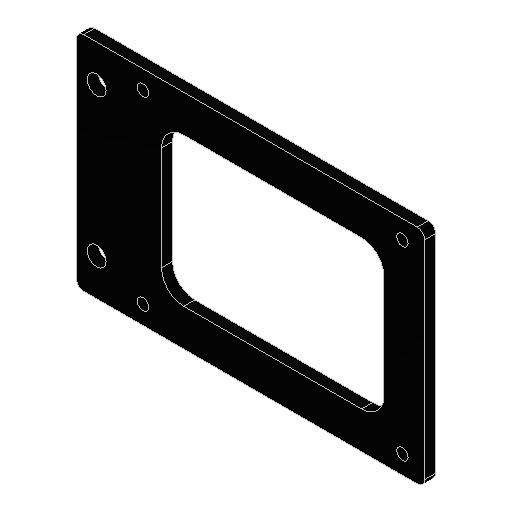
# Autodesk Inventor part: PCB plate
Saved by Autodesk Inventor 2022.4 (Build 264492000, 492)
## iProperties
Category: -
Company: Universiteit van Amsterdam
Created: 2023-09-04
Part Number: PCB plate
Material: ALMg4,5Mn-5083-(D54S)
Document SubType Name: Modeling
Designer: Ronald Hassing
Density: 2.66 g/cm^3
Appearance: Aluminum - Flat(2)
User Status: Work in Progress
Author: Ronald Hassing
Revision Number: A
Autodesk Inventor part; units mm, degrees
ref_plane "YZ Plane" through (0, 0, 0) normal (1, 0, 0) x (0, 1, 0)
ref_plane "XZ Plane" through (0, 0, 0) normal (0, 1, 0) x (-1, 0, 0)
ref_plane "XY Plane" through (0, 0, 0) normal (0, 0, 1) x (1, 0, 0)
sketch "Sketch1" plane through (0, 0, 0) normal (0, 0, 1) x (1, 0, 0)
  line L0 (0, 42) -> (0, -42) construction
  line L1 (-71.8, 0) -> (59.8, 0) construction
  line L2 (-39, -29) -> (39, -29) construction
  line L3 (39, -29) -> (39, 29) construction
  line L4 (39, 29) -> (-39, 29) construction
  line L5 (-39, 29) -> (-39, -29) construction
  line L6 (-39, -29) -> (39, 29) construction
  line L7 (39, -29) -> (-39, 29) construction
  line L8 (-35, -25) -> (35, -25) construction
  line L9 (35, -25) -> (35, 25) construction
  line L10 (35, 25) -> (-35, 25) construction
  line L11 (-35, 25) -> (-35, -25) construction
  line L12 (-35, -25) -> (35, 25) construction
  line L13 (35, -25) -> (-35, 25) construction
  circle A0 centre (-35, 25) radius 1.55
  circle A1 centre (-35, -25) radius 1.55
  circle A2 centre (35, -25) radius 1.55
  circle A3 centre (35, 25) radius 1.55
  line L14 (-53, 30) -> (41, 30)
  line L15 (41, 30) -> (41, -30)
  line L16 (41, -30) -> (-53, -30)
  line L17 (-53, -30) -> (-53, 30)
  line L18 (-30, -20) -> (30, -20)
  line L19 (30, -20) -> (30, 20)
  line L20 (30, 20) -> (-30, 20)
  line L21 (-30, 20) -> (-30, -20)
  line L22 (-30, -20) -> (30, 20) construction
  line L23 (30, -20) -> (-30, 20) construction
  circle A4 centre (-47.5, 20) radius 2.55
  circle A5 centre (-47.5, -20) radius 2.55
  point P0 (0, 0)
  point P1 (-53, 0)
  point P2 (-39, 0)
  dimension "d4" = 58
  dimension "d5" = 78
  dimension "d6" = 4
  dimension "d7" = 50
  dimension "d8" = 3.1
  dimension "d9" = 14
  dimension "d10" = 60
  dimension "d12" = 40
  dimension "d13" = 60
  dimension "d16" = 2
  dimension "d17" = 5.1
  dimension "d18" = 20
  dimension "d19" = 5.5
  dimension "d20" = 20
  constraints: 44 end point, 8 midpoint, 8 parallel, 6 centre point, 4 coincident, 4 equal radius, 4 horizontal, 4 perpendicular, 1 horizontal alignment, 1 vertical alignment
  measures "d4" distance of L2.end L3.end
  measures "d5" distance of L3.end L4.end
  measures "d6" distance between parallel lines of L5 L11
  measures "d7" distance of L8.end L9.end
  measures "d8" diameter of A3
  measures "d9" distance between parallel lines of L17 L5
  measures "d10" distance of L16.end L14.start
  measures "d12" distance between parallel lines of L18 L20
  measures "d13" distance between parallel lines of L21 L19
  measures "d16" distance between parallel lines of L15 L3
  measures "d17" diameter of A4
  measures "d18" vertical distance of point (-53, 0) A4.centre
  measures "d19" distance from line of L17 A4.centre
  measures "d20" vertical distance of A5.centre point (-53, 0)
extrude "Extrusion3" add sketch "Sketch1" along normal blind 3
fillet "Fillet1" radius 6 4 edges at (-30, 20, 1.5) (-30, -20, 1.5) (30, -20, 1.5) (30, 20, 1.5)
fillet "Fillet2" radius 2 4 edges at (41, 30, 1.5) (-53, 30, 1.5) (-53, -30, 1.5) (41, -30, 1.5)
body "Solid3"
